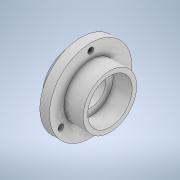
# Autodesk Inventor part: capa da engrenagem
Saved by Autodesk Inventor 2022.1 (Build 261234020, 234B)
## iProperties
Created: 2023-10-20
Part Number: capa da engrenagem
Material: Generic
Document SubType Name: Modeling
Designer: SENAI
Density: 1 g/cm^3
Appearance: Default
Author: SENAI
Autodesk Inventor part; units mm, degrees
ref_plane "YZ Plane" through (0, 0, 0) normal (1, 0, 0) x (0, 1, 0)
ref_plane "XZ Plane" through (0, 0, 0) normal (0, 1, 0) x (-1, 0, 0)
ref_plane "XY Plane" through (0, 0, 0) normal (0, 0, 1) x (1, 0, 0)
sketch "Sketch1" plane through (0, 0, 0) normal (0, 0, 1) x (1, 0, 0)
  line L0 (0, 0) -> (0, 32.5)
  line L1 (0, 32.5) -> (13, 32.5)
  line L2 (13, 32.5) -> (13, 48.5)
  line L3 (13, 48.5) -> (24.3, 48.5)
  line L4 (24.3, 48.5) -> (24.3, 31.5)
  line L5 (24.3, 31.5) -> (46.9, 31.5)
  line L6 (46.9, 31.5) -> (46.9, 0)
  line L7 (0, 0) -> (46.9, 0)
  dimension "d0" = 32.5
  dimension "d1" = 13
  dimension "d2" = 16
  dimension "d3" = 11.3
  dimension "d4" = 17
  dimension "d5" = 22.6
  constraints: 16 end point, 3 horizontal, 3 perpendicular, 2 vertical
  measures "d0" distance of L0.start L0.end
  measures "d1" distance of L0.end L1.end
  measures "d2" distance of L1.end L2.end
  measures "d3" distance of L2.end L3.end
  measures "d4" distance of L3.end L4.end
  measures "d5" distance of L4.end L5.end
revolve "Revolution1" add sketch "Sketch1" angle 360 about axis through (0, 0, 0) along (1, 0, 0)
sketch "Sketch2" plane through (13, 0, 0) normal (-1, 0, 0) x (0, 0, 1)
  circle A0 centre (0, 0) radius 32.5 projected
  circle A1 centre (0, 0) radius 48.5 projected
  circle A2 centre (0, 40.5) radius 3.5
  circle A3 centre (35.074, -20.25) radius 3.5
  circle A4 centre (-35.074, -20.25) radius 3.5
  dimension "d11" = 7
  dimension "d12" = 7
  dimension "d13" = 7
  constraints: 3 centre point, 3 coincident
  measures "d11" diameter of A2
  measures "d12" diameter of A3
  measures "d13" diameter of A4
extrude "Extrusion1" cut sketch "Sketch2" against normal through all contours A2 | A3 | A4
sketch "Sketch3" plane through (0, 0, 0) normal (-1, 0, 0) x (0, 0, 1)
  circle A0 centre (0, 0) radius 17.5
  dimension "d16" = 35
  constraints: 1 centre point, 1 coincident
  measures "d16" diameter of A0
sketch "Sketch4" plane through (0, 0, 0) normal (-1, 0, 0) x (0, 0, 1)
  point P0 (0, 0)
extrude "Extrusion2" cut sketch "Sketch3" against normal through all
sketch "Sketch5" plane through (46.9, 0, 0) normal (1, 0, 0) x (0, 0, -1)
  circle A0 centre (0, 0) radius 31.5 projected
  circle A1 centre (0, 0) radius 26.2
  constraints: 1 centre point, 1 coincident
extrude "Extrusion3" cut sketch "Sketch5" against normal blind 22.5 contours A1
body "Solid1"
